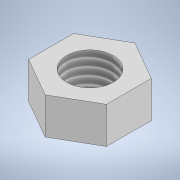
# Autodesk Inventor part: 29_Dado_M6
Saved by Autodesk Inventor 2020.2 (Build 242310000, 310)
## iProperties
Created: 2019-12-29
Part Number: 29_Dado_M6
Material: Acciaio inox AISI 316
Document SubType Name: Modeling
Designer: socci
Density: 8 g/cm^3
Appearance: Default(1)
Author: socci
Autodesk Inventor part; units mm, degrees
ref_plane "YZ Plane" through (0, 0, 0) normal (1, 0, 0) x (0, 1, 0)
ref_plane "XZ Plane" through (0, 0, 0) normal (0, 1, 0) x (-1, 0, 0)
ref_plane "XY Plane" through (0, 0, 0) normal (0, 0, 1) x (1, 0, 0)
sketch "Schizzo1" plane through (0, 0, 0) normal (0, 1, 0) x (-1, 0, 0)
  circle A0 centre (0, 0) radius 5 construction
  line L0 (5, -2.8868) -> (0, -5.7735)
  line L1 (0, -5.7735) -> (-5, -2.8868)
  line L2 (-5, -2.8868) -> (-5, 2.8868)
  line L3 (-5, 2.8868) -> (0, 5.7735)
  line L4 (0, 5.7735) -> (5, 2.8868)
  line L5 (5, 2.8868) -> (5, -2.8868)
  point P0 (5, 0)
  dimension "d0" = 10
  constraints: 12 end point, 2 coincident, 1 horizontal alignment, 1 midpoint, 15 other
extrude "Estrusione1" add sketch "Schizzo1" along normal blind 4.7
sketch "Schizzo2" plane through (0, 4.7, 0) normal (0, 1, 0) x (1, 0, 0)
  circle A0 centre (0, 0) radius 3
  dimension "d3" = 6
  constraints: 1 centre point, 1 coincident
  measures "d3" diameter of A0
extrude "Estrusione2" cut sketch "Schizzo2" against normal blind 4.7
thread "Filettatura1" size "M6x1" class "6H" standard "ANSI Metric M Profile" length 100
